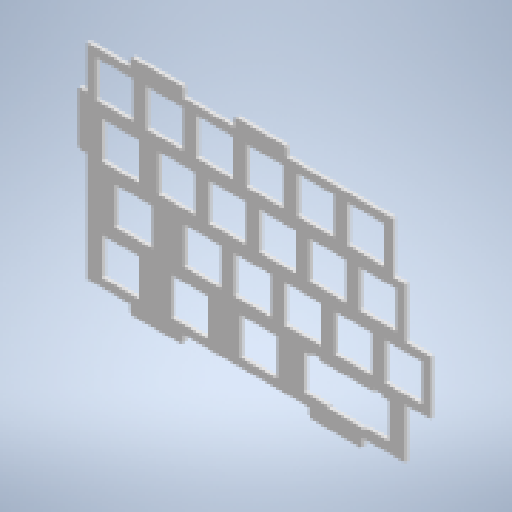
# Autodesk Inventor part: Plate_Left
Saved by Autodesk Inventor 2023 (Build 270158000, 158)
## iProperties
Created: 2022-11-13
Part Number: Plate_Left
Material: Generic
Document SubType Name: Modeling
Designer: reide
Density: 1 g/cm^3
Appearance: Default
Author: reide
Autodesk Inventor part; units mm, degrees
ref_plane "YZ Plane" through (0, 0, 0) normal (1, 0, 0) x (0, 1, 0)
ref_plane "XZ Plane" through (0, 0, 0) normal (0, 1, 0) x (-1, 0, 0)
ref_plane "XY Plane" through (0, 0, 0) normal (0, 0, 1) x (1, 0, 0)
sketch "Sketch1" plane through (0, 0, 0) normal (0, 0, 1) x (1, 0, 0)
  line L0 (115.8, 77.7) -> (0, 77.7)
  line L1 (0, 77.7) -> (0, 0)
  line L2 (0, 0) -> (120.562, 0)
  line L3 (120.562, 19.05) -> (120.562, 0)
  line L4 (130.0875, 19.05) -> (120.562, 19.05)
  line L5 (130.0875, 39.6) -> (130.0875, 19.05)
  line L6 (120.5625, 39.6) -> (130.0875, 39.6)
  line L7 (120.5625, 58.65) -> (120.5625, 39.6)
  line L8 (115.8, 58.65) -> (120.5625, 58.65)
  line L9 (115.8, 77.7) -> (115.8, 58.65)
  line L10 (10.4187, 22.325) -> (10.4187, 36.325)
  line L11 (10.4187, 36.325) -> (24.4187, 36.325)
  line L12 (24.4187, 36.325) -> (24.4187, 22.325)
  line L13 (24.4187, 22.325) -> (10.4187, 22.325)
  line L14 (58.0437, 3.275) -> (58.0437, 17.275)
  line L15 (58.0437, 17.275) -> (72.0437, 17.275)
  line L16 (72.0437, 17.275) -> (72.0437, 3.275)
  line L17 (72.0437, 3.275) -> (58.0437, 3.275)
  line L18 (31.85, 3.275) -> (31.85, 17.275)
  line L19 (31.85, 17.275) -> (45.85, 17.275)
  line L20 (45.85, 17.275) -> (45.85, 3.275)
  line L21 (45.85, 3.275) -> (31.85, 3.275)
  line L22 (5.6562, 3.275) -> (5.6562, 17.275)
  line L23 (5.6562, 17.275) -> (19.6562, 17.275)
  line L24 (19.6562, 17.275) -> (19.6562, 3.275)
  line L25 (19.6562, 3.275) -> (5.6562, 3.275)
  line L26 (5.6562, 41.375) -> (5.6562, 55.375)
  line L27 (5.6562, 55.375) -> (19.6562, 55.375)
  line L28 (19.6562, 55.375) -> (19.6562, 41.375)
  line L29 (19.6562, 41.375) -> (5.6562, 41.375)
  line L30 (112.8125, 22.325) -> (112.8125, 36.325)
  line L31 (112.8125, 36.325) -> (126.8125, 36.325)
  line L32 (126.8125, 36.325) -> (126.8125, 22.325)
  line L33 (126.8125, 22.325) -> (112.8125, 22.325)
  line L34 (93.7625, 22.325) -> (93.7625, 36.325)
  line L35 (93.7625, 36.325) -> (107.7625, 36.325)
  line L36 (107.7625, 36.325) -> (107.7625, 22.325)
  line L37 (107.7625, 22.325) -> (93.7625, 22.325)
  line L38 (74.7125, 22.325) -> (74.7125, 36.325)
  line L39 (74.7125, 36.325) -> (88.7125, 36.325)
  line L40 (88.7125, 36.325) -> (88.7125, 22.325)
  line L41 (88.7125, 22.325) -> (74.7125, 22.325)
  line L42 (55.6625, 22.325) -> (55.6625, 36.325)
  line L43 (55.6625, 36.325) -> (69.6625, 36.325)
  line L44 (69.6625, 36.325) -> (69.6625, 22.325)
  line L45 (69.6625, 22.325) -> (55.6625, 22.325)
  line L46 (36.6125, 22.325) -> (36.6125, 36.325)
  line L47 (36.6125, 36.325) -> (50.6125, 36.325)
  line L48 (50.6125, 36.325) -> (50.6125, 22.325)
  line L49 (50.6125, 22.325) -> (36.6125, 22.325)
  line L50 (103.2875, 41.375) -> (103.2875, 55.375)
  line L51 (103.2875, 55.375) -> (117.2875, 55.375)
  line L52 (117.2875, 55.375) -> (117.2875, 41.375)
  line L53 (117.2875, 41.375) -> (103.2875, 41.375)
  line L54 (84.2375, 41.375) -> (84.2375, 55.375)
  line L55 (84.2375, 55.375) -> (98.2375, 55.375)
  line L56 (98.2375, 55.375) -> (98.2375, 41.375)
  line L57 (98.2375, 41.375) -> (84.2375, 41.375)
  line L58 (65.1875, 41.375) -> (65.1875, 55.375)
  line L59 (65.1875, 55.375) -> (79.1875, 55.375)
  line L60 (79.1875, 55.375) -> (79.1875, 41.375)
  line L61 (79.1875, 41.375) -> (65.1875, 41.375)
  line L62 (46.1375, 41.375) -> (46.1375, 55.375)
  line L63 (46.1375, 55.375) -> (60.1375, 55.375)
  line L64 (60.1375, 55.375) -> (60.1375, 41.375)
  line L65 (60.1375, 41.375) -> (46.1375, 41.375)
  line L66 (27.0875, 41.375) -> (27.0875, 55.375)
  line L67 (27.0875, 55.375) -> (41.0875, 55.375)
  line L68 (41.0875, 55.375) -> (41.0875, 41.375)
  line L69 (41.0875, 41.375) -> (27.0875, 41.375)
  line L70 (98.525, 60.425) -> (98.525, 74.425)
  line L71 (98.525, 74.425) -> (112.525, 74.425)
  line L72 (112.525, 74.425) -> (112.525, 60.425)
  line L73 (112.525, 60.425) -> (98.525, 60.425)
  line L74 (79.475, 60.425) -> (79.475, 74.425)
  line L75 (79.475, 74.425) -> (93.475, 74.425)
  line L76 (93.475, 74.425) -> (93.475, 60.425)
  line L77 (93.475, 60.425) -> (79.475, 60.425)
  line L78 (60.425, 60.425) -> (60.425, 74.425)
  line L79 (60.425, 74.425) -> (74.425, 74.425)
  line L80 (74.425, 74.425) -> (74.425, 60.425)
  line L81 (74.425, 60.425) -> (60.425, 60.425)
  line L82 (41.375, 60.425) -> (41.375, 74.425)
  line L83 (41.375, 74.425) -> (55.375, 74.425)
  line L84 (55.375, 74.425) -> (55.375, 60.425)
  line L85 (55.375, 60.425) -> (41.375, 60.425)
  line L86 (22.325, 60.425) -> (22.325, 74.425)
  line L87 (22.325, 74.425) -> (36.325, 74.425)
  line L88 (36.325, 74.425) -> (36.325, 60.425)
  line L89 (36.325, 60.425) -> (22.325, 60.425)
  line L90 (3.275, 60.425) -> (3.275, 74.425)
  line L91 (3.275, 74.425) -> (17.275, 74.425)
  line L92 (17.275, 74.425) -> (17.275, 60.425)
  line L93 (17.275, 60.425) -> (3.275, 60.425)
  line L94 (88.1304, 17.275) -> (108.6315, 17.275)
  line L95 (108.6315, 17.275) -> (108.6315, 18.2451)
  line L96 (108.6315, 18.2451) -> (111.9306, 18.2451)
  line L97 (111.9306, 18.2451) -> (111.9306, 17.275)
  line L98 (111.9306, 17.275) -> (114.4058, 17.275)
  line L99 (114.4058, 17.275) -> (114.4059, 17.0334)
  line L100 (114.4059, 17.0334) -> (114.4058, 3.9957)
  line L101 (114.4058, 3.9957) -> (106.9062, 3.9957)
  line L102 (106.9062, 3.9957) -> (105.3807, 3.9957)
  line L103 (105.3807, 3.9957) -> (105.3807, 3.2757)
  line L104 (105.3807, 3.2757) -> (91.3812, 3.2757)
  line L105 (91.3812, 3.2757) -> (91.3812, 3.9957)
  line L106 (91.3812, 3.9957) -> (82.3562, 3.9957)
  line L107 (82.3562, 3.9957) -> (82.3562, 17.0464)
  line L108 (82.3562, 17.0464) -> (82.3562, 17.275)
  line L109 (82.3562, 17.275) -> (84.8314, 17.275)
  line L110 (84.8314, 17.275) -> (84.8314, 18.2451)
  line L111 (84.8314, 18.2451) -> (88.1304, 18.2451)
  line L112 (88.1304, 18.2451) -> (88.1304, 17.275)
  point P0 (0.75, 76.95)
  constraints: 226 end point
extrude "Extrusion1" add sketch "Sketch1" along normal blind 1.4
sketch "Sketch2" plane through (0, 0, 1.4) normal (0, 0, 1) x (1, 0, 0)
  line L0 (19.6562, 41.375) -> (5.6562, 41.375) projected
  line L1 (0, 77.7) -> (0, 0) projected
  line L2 (0, 41.375) -> (0, 61.375)
  line L3 (0, 61.375) -> (-3.5, 61.375)
  line L4 (-3.5, 61.375) -> (-3.5, 41.375)
  line L5 (-3.5, 41.375) -> (0, 41.375)
  arc A0 (77.3, 76.2) -> (81.3, 80.2) centre (77.3, 80.2) ccw projected
  line L6 (1.25, 76.2) -> (77.3, 76.2) projected
  line L7 (1.25, 41.0243) -> (1.25, 76.2) projected
  line L8 (-0.25, 41.0243) -> (1.25, 41.0243) projected
  line L9 (-0.25, 41.0243) -> (-0.25, 33.75) projected
  line L10 (-0.25, 33.75) -> (-1.25, 33.75) projected
  line L11 (-1.25, 33.75) -> (-1.25, 35.75) projected
  line L12 (-1.25, 35.75) -> (-5.25, 35.75) projected
  line L13 (-5.25, 35.75) -> (-5.25, 81.45) projected
  arc A1 (-2.25, 84.45) -> (-5.25, 81.45) centre (-2.25, 81.45) ccw projected
  line L14 (85.05, 84.45) -> (-2.25, 84.45) projected
  line L15 (85.05, 83.45) -> (85.05, 84.45) projected
  line L16 (81.3, 83.45) -> (85.05, 83.45) projected
  line L17 (81.3, 80.2) -> (81.3, 83.45) projected
  circle A2 centre (63.044, 80.2) radius 1.5 projected
  circle A3 centre (-1, 80.2) radius 1.5 projected
  circle A4 centre (-1.75, 49.45) radius 1.5 projected
  line L18 (117.025, 56.875) -> (117.7875, 56.875) projected
  line L19 (117.7875, 56.875) -> (117.7875, 41.825) projected
  arc A5 (117.7875, 41.825) -> (121.7875, 37.825) centre (121.7875, 41.825) ccw projected
  line L20 (121.7875, 37.825) -> (116.8125, 37.825) projected
  line L21 (116.8125, 37.825) -> (116.8125, 36.325) projected
  line L22 (116.8125, 36.325) -> (112.8125, 36.325) projected
  line L23 (112.8125, 36.325) -> (112.8125, 22.325) projected
  line L24 (112.8125, 22.325) -> (107.7625, 22.325) projected
  line L25 (107.7625, 22.325) -> (107.7625, 36.325) projected
  line L26 (107.7625, 36.325) -> (103.7625, 36.325) projected
  line L27 (103.7625, 36.325) -> (103.7625, 37.825) projected
  line L28 (103.7625, 37.825) -> (97.7625, 37.825) projected
  line L29 (97.7625, 37.825) -> (97.7625, 36.325) projected
  line L30 (97.7625, 36.325) -> (93.7625, 36.325) projected
  line L31 (93.7625, 36.325) -> (93.7625, 22.325) projected
  line L32 (93.7625, 22.325) -> (88.7125, 22.325) projected
  line L33 (88.7125, 22.325) -> (88.7125, 36.325) projected
  line L34 (88.7125, 36.325) -> (84.7125, 36.325) projected
  line L35 (84.7125, 36.325) -> (84.7125, 37.825) projected
  line L36 (84.7125, 37.825) -> (78.7125, 37.825) projected
  line L37 (78.7125, 37.825) -> (78.7125, 36.325) projected
  line L38 (78.7125, 36.325) -> (74.7125, 36.325) projected
  line L39 (74.7125, 36.325) -> (74.7125, 22.325) projected
  line L40 (74.7125, 22.325) -> (78.7125, 22.325) projected
  line L41 (78.7125, 22.325) -> (78.7125, 20.825) projected
  line L42 (78.7125, 20.825) -> (83.1062, 20.825) projected
  line L43 (83.1062, 20.825) -> (83.1062, 17.275) projected
  line L44 (83.1062, 17.275) -> (82.3562, 17.275) projected
  line L45 (82.3562, 17.275) -> (82.3562, 17.0464) projected
  line L46 (82.3562, 17.0464) -> (82.3562, 3.9957) projected
  line L47 (82.3562, 3.9957) -> (83.1062, 3.9957) projected
  line L48 (83.1062, 3.9957) -> (83.1062, 1.5) projected
  line L49 (83.1062, 1.5) -> (1.25, 1.5) projected
  line L50 (1.25, 1.5) -> (1.25, 18.4694) projected
  line L51 (1.25, 18.4694) -> (-0.25, 18.4694) projected
  line L52 (-0.25, 41.0243) -> (-0.25, 18.4694) projected
  line L53 (-0.25, 41.0243) -> (1.25, 41.0243) projected
  line L54 (1.25, 41.0243) -> (1.25, 76.2) projected
  line L55 (1.25, 76.2) -> (77.3, 76.2) projected
  arc A6 (77.3, 76.2) -> (81.3, 80.2) centre (77.3, 80.2) ccw projected
  line L56 (81.3, 80.2) -> (81.3, 83.45) projected
  line L57 (81.3, 83.45) -> (99.3, 83.45) projected
  line L58 (99.3, 83.45) -> (99.3, 80.2) projected
  arc A7 (99.3, 80.2) -> (103.3, 76.2) centre (103.3, 80.2) ccw projected
  line L59 (103.3, 76.2) -> (113.025, 76.2) projected
  line L60 (113.025, 76.2) -> (113.025, 60.875) projected
  arc A8 (113.025, 60.875) -> (117.025, 56.875) centre (117.025, 60.875) ccw projected
  line L61 (113.2875, 56.875) -> (107.2875, 56.875) projected
  line L62 (107.2875, 56.875) -> (107.2875, 55.375) projected
  line L63 (107.2875, 55.375) -> (103.2875, 55.375) projected
  line L64 (103.2875, 55.375) -> (103.2875, 41.375) projected
  line L65 (103.2875, 41.375) -> (107.2875, 41.375) projected
  line L66 (107.2875, 41.375) -> (107.2875, 39.875) projected
  line L67 (107.2875, 39.875) -> (113.2875, 39.875) projected
  line L68 (113.2875, 39.875) -> (113.2875, 41.375) projected
  line L69 (113.2875, 41.375) -> (117.2875, 41.375) projected
  line L70 (117.2875, 41.375) -> (117.2875, 55.375) projected
  line L71 (117.2875, 55.375) -> (113.2875, 55.375) projected
  line L72 (113.2875, 55.375) -> (113.2875, 56.875) projected
  line L73 (13.275, 58.925) -> (13.275, 60.425) projected
  line L74 (13.275, 60.425) -> (17.275, 60.425) projected
  line L75 (17.275, 60.425) -> (17.275, 74.425) projected
  line L76 (17.275, 74.425) -> (13.275, 74.425) projected
  line L77 (13.275, 74.425) -> (13.275, 75.925) projected
  line L78 (13.275, 75.925) -> (7.275, 75.925) projected
  line L79 (7.275, 75.925) -> (7.275, 74.425) projected
  line L80 (7.275, 74.425) -> (3.275, 74.425) projected
  line L81 (3.275, 74.425) -> (3.275, 60.425) projected
  line L82 (3.275, 60.425) -> (7.275, 60.425) projected
  line L83 (7.275, 60.425) -> (7.275, 58.925) projected
  line L84 (7.275, 58.925) -> (13.275, 58.925) projected
  line L85 (32.325, 58.925) -> (32.325, 60.425) projected
  line L86 (32.325, 60.425) -> (36.325, 60.425) projected
  line L87 (36.325, 60.425) -> (36.325, 74.425) projected
  line L88 (36.325, 74.425) -> (32.325, 74.425) projected
  line L89 (32.325, 74.425) -> (32.325, 75.925) projected
  line L90 (32.325, 75.925) -> (26.325, 75.925) projected
  line L91 (26.325, 75.925) -> (26.325, 74.425) projected
  line L92 (26.325, 74.425) -> (22.325, 74.425) projected
  line L93 (22.325, 74.425) -> (22.325, 60.425) projected
  line L94 (22.325, 60.425) -> (26.325, 60.425) projected
  line L95 (26.325, 60.425) -> (26.325, 58.925) projected
  line L96 (26.325, 58.925) -> (32.325, 58.925) projected
  line L97 (51.375, 58.925) -> (51.375, 60.425) projected
  line L98 (51.375, 60.425) -> (55.375, 60.425) projected
  line L99 (55.375, 60.425) -> (55.375, 74.425) projected
  line L100 (55.375, 74.425) -> (51.375, 74.425) projected
  line L101 (51.375, 74.425) -> (51.375, 75.925) projected
  line L102 (51.375, 75.925) -> (45.375, 75.925) projected
  line L103 (45.375, 75.925) -> (45.375, 74.425) projected
  line L104 (45.375, 74.425) -> (41.375, 74.425) projected
  line L105 (41.375, 74.425) -> (41.375, 60.425) projected
  line L106 (41.375, 60.425) -> (45.375, 60.425) projected
  line L107 (45.375, 60.425) -> (45.375, 58.925) projected
  line L108 (45.375, 58.925) -> (51.375, 58.925) projected
  line L109 (70.425, 58.925) -> (70.425, 60.425) projected
  line L110 (70.425, 60.425) -> (74.425, 60.425) projected
  line L111 (74.425, 60.425) -> (74.425, 74.425) projected
  line L112 (74.425, 74.425) -> (70.425, 74.425) projected
  line L113 (70.425, 74.425) -> (70.425, 75.925) projected
  line L114 (70.425, 75.925) -> (64.425, 75.925) projected
  line L115 (64.425, 75.925) -> (64.425, 74.425) projected
  line L116 (64.425, 74.425) -> (60.425, 74.425) projected
  line L117 (60.425, 74.425) -> (60.425, 60.425) projected
  line L118 (60.425, 60.425) -> (64.425, 60.425) projected
  line L119 (64.425, 60.425) -> (64.425, 58.925) projected
  line L120 (64.425, 58.925) -> (70.425, 58.925) projected
  line L121 (89.475, 58.925) -> (89.475, 60.425) projected
  line L122 (89.475, 60.425) -> (93.475, 60.425) projected
  line L123 (93.475, 60.425) -> (93.475, 74.425) projected
  line L124 (93.475, 74.425) -> (89.475, 74.425) projected
  line L125 (89.475, 74.425) -> (89.475, 75.925) projected
  line L126 (89.475, 75.925) -> (83.475, 75.925) projected
  line L127 (83.475, 75.925) -> (83.475, 74.425) projected
  line L128 (83.475, 74.425) -> (79.475, 74.425) projected
  line L129 (79.475, 74.425) -> (79.475, 60.425) projected
  line L130 (79.475, 60.425) -> (83.475, 60.425) projected
  line L131 (83.475, 60.425) -> (83.475, 58.925) projected
  line L132 (83.475, 58.925) -> (89.475, 58.925) projected
  line L133 (108.525, 58.925) -> (108.525, 60.425) projected
  line L134 (108.525, 60.425) -> (112.525, 60.425) projected
  line L135 (112.525, 60.425) -> (112.525, 74.425) projected
  line L136 (112.525, 74.425) -> (108.525, 74.425) projected
  line L137 (108.525, 74.425) -> (108.525, 75.925) projected
  line L138 (108.525, 75.925) -> (102.525, 75.925) projected
  line L139 (102.525, 75.925) -> (102.525, 74.425) projected
  line L140 (102.525, 74.425) -> (98.525, 74.425) projected
  line L141 (98.525, 74.425) -> (98.525, 60.425) projected
  line L142 (98.525, 60.425) -> (102.525, 60.425) projected
  line L143 (102.525, 60.425) -> (102.525, 58.925) projected
  line L144 (102.525, 58.925) -> (108.525, 58.925) projected
  line L145 (37.0875, 39.875) -> (37.0875, 41.375) projected
  line L146 (37.0875, 41.375) -> (41.0875, 41.375) projected
  line L147 (41.0875, 41.375) -> (41.0875, 55.375) projected
  line L148 (41.0875, 55.375) -> (37.0875, 55.375) projected
  line L149 (37.0875, 55.375) -> (37.0875, 56.875) projected
  line L150 (37.0875, 56.875) -> (31.0875, 56.875) projected
  line L151 (31.0875, 56.875) -> (31.0875, 55.375) projected
  line L152 (31.0875, 55.375) -> (27.0875, 55.375) projected
  line L153 (27.0875, 55.375) -> (27.0875, 41.375) projected
  line L154 (27.0875, 41.375) -> (31.0875, 41.375) projected
  line L155 (31.0875, 41.375) -> (31.0875, 39.875) projected
  line L156 (31.0875, 39.875) -> (37.0875, 39.875) projected
  line L157 (50.1375, 56.875) -> (50.1375, 55.375) projected
  line L158 (50.1375, 55.375) -> (46.1375, 55.375) projected
  line L159 (46.1375, 55.375) -> (46.1375, 41.375) projected
  line L160 (46.1375, 41.375) -> (50.1375, 41.375) projected
  line L161 (50.1375, 41.375) -> (50.1375, 39.875) projected
  line L162 (50.1375, 39.875) -> (56.1375, 39.875) projected
  line L163 (56.1375, 39.875) -> (56.1375, 41.375) projected
  line L164 (56.1375, 41.375) -> (60.1375, 41.375) projected
  line L165 (60.1375, 41.375) -> (60.1375, 55.375) projected
  line L166 (60.1375, 55.375) -> (56.1375, 55.375) projected
  line L167 (56.1375, 55.375) -> (56.1375, 56.875) projected
  line L168 (56.1375, 56.875) -> (50.1375, 56.875) projected
  line L169 (69.1875, 56.875) -> (69.1875, 55.375) projected
  line L170 (69.1875, 55.375) -> (65.1875, 55.375) projected
  line L171 (65.1875, 55.375) -> (65.1875, 41.375) projected
  line L172 (65.1875, 41.375) -> (69.1875, 41.375) projected
  line L173 (69.1875, 41.375) -> (69.1875, 39.875) projected
  line L174 (69.1875, 39.875) -> (75.1875, 39.875) projected
  line L175 (75.1875, 39.875) -> (75.1875, 41.375) projected
  line L176 (75.1875, 41.375) -> (79.1875, 41.375) projected
  line L177 (79.1875, 41.375) -> (79.1875, 55.375) projected
  line L178 (79.1875, 55.375) -> (75.1875, 55.375) projected
  line L179 (75.1875, 55.375) -> (75.1875, 56.875) projected
  line L180 (75.1875, 56.875) -> (69.1875, 56.875) projected
  line L181 (88.2375, 56.875) -> (88.2375, 55.375) projected
  line L182 (88.2375, 55.375) -> (84.2375, 55.375) projected
  line L183 (84.2375, 55.375) -> (84.2375, 41.375) projected
  line L184 (84.2375, 41.375) -> (88.2375, 41.375) projected
  line L185 (88.2375, 41.375) -> (88.2375, 39.875) projected
  line L186 (88.2375, 39.875) -> (94.2375, 39.875) projected
  line L187 (94.2375, 39.875) -> (94.2375, 41.375) projected
  line L188 (94.2375, 41.375) -> (98.2375, 41.375) projected
  line L189 (98.2375, 41.375) -> (98.2375, 55.375) projected
  line L190 (98.2375, 55.375) -> (94.2375, 55.375) projected
  line L191 (94.2375, 55.375) -> (94.2375, 56.875) projected
  line L192 (94.2375, 56.875) -> (88.2375, 56.875) projected
  line L193 (46.6125, 20.825) -> (46.6125, 22.325) projected
  line L194 (46.6125, 22.325) -> (50.6125, 22.325) projected
  line L195 (50.6125, 22.325) -> (50.6125, 36.325) projected
  line L196 (50.6125, 36.325) -> (46.6125, 36.325) projected
  line L197 (46.6125, 36.325) -> (46.6125, 37.825) projected
  line L198 (46.6125, 37.825) -> (40.6125, 37.825) projected
  line L199 (40.6125, 37.825) -> (40.6125, 36.325) projected
  line L200 (40.6125, 36.325) -> (36.6125, 36.325) projected
  line L201 (36.6125, 36.325) -> (36.6125, 22.325) projected
  line L202 (36.6125, 22.325) -> (40.6125, 22.325) projected
  line L203 (40.6125, 22.325) -> (40.6125, 20.825) projected
  line L204 (40.6125, 20.825) -> (46.6125, 20.825) projected
  line L205 (65.6625, 20.825) -> (65.6625, 22.325) projected
  line L206 (65.6625, 22.325) -> (69.6625, 22.325) projected
  line L207 (69.6625, 22.325) -> (69.6625, 36.325) projected
  line L208 (69.6625, 36.325) -> (65.6625, 36.325) projected
  line L209 (65.6625, 36.325) -> (65.6625, 37.825) projected
  line L210 (65.6625, 37.825) -> (59.6625, 37.825) projected
  line L211 (59.6625, 37.825) -> (59.6625, 36.325) projected
  line L212 (59.6625, 36.325) -> (55.6625, 36.325) projected
  line L213 (55.6625, 36.325) -> (55.6625, 22.325) projected
  line L214 (55.6625, 22.325) -> (59.6625, 22.325) projected
  line L215 (59.6625, 22.325) -> (59.6625, 20.825) projected
  line L216 (59.6625, 20.825) -> (65.6625, 20.825) projected
  line L217 (15.6562, 39.875) -> (15.6562, 41.375) projected
  line L218 (15.6562, 41.375) -> (19.6562, 41.375) projected
  line L219 (19.6562, 41.375) -> (19.6562, 55.375) projected
  line L220 (19.6562, 55.375) -> (15.6562, 55.375) projected
  line L221 (15.6562, 55.375) -> (15.6562, 56.875) projected
  line L222 (15.6562, 56.875) -> (9.6562, 56.875) projected
  line L223 (9.6562, 56.875) -> (9.6562, 55.375) projected
  line L224 (9.6562, 55.375) -> (5.6562, 55.375) projected
  line L225 (5.6562, 55.375) -> (5.6562, 41.375) projected
  line L226 (5.6562, 41.375) -> (9.6562, 41.375) projected
  line L227 (9.6562, 41.375) -> (9.6562, 39.875) projected
  line L228 (9.6562, 39.875) -> (15.6562, 39.875) projected
  line L229 (20.4187, 20.825) -> (20.4187, 22.325) projected
  line L230 (20.4187, 22.325) -> (24.4187, 22.325) projected
  line L231 (24.4187, 22.325) -> (24.4187, 36.325) projected
  line L232 (24.4187, 36.325) -> (20.4187, 36.325) projected
  line L233 (20.4187, 36.325) -> (20.4187, 37.825) projected
  line L234 (20.4187, 37.825) -> (14.4187, 37.825) projected
  line L235 (14.4187, 37.825) -> (14.4187, 36.325) projected
  line L236 (14.4187, 36.325) -> (10.4187, 36.325) projected
  line L237 (10.4187, 36.325) -> (10.4187, 22.325) projected
  line L238 (10.4187, 22.325) -> (14.4187, 22.325) projected
  line L239 (14.4187, 22.325) -> (14.4187, 20.825) projected
  line L240 (14.4187, 20.825) -> (20.4187, 20.825) projected
  line L241 (15.6562, 1.775) -> (15.6562, 3.275) projected
  line L242 (15.6562, 3.275) -> (19.6562, 3.275) projected
  line L243 (19.6562, 3.275) -> (19.6562, 17.275) projected
  line L244 (19.6562, 17.275) -> (15.6562, 17.275) projected
  line L245 (15.6562, 17.275) -> (15.6562, 18.775) projected
  line L246 (15.6562, 18.775) -> (9.6562, 18.775) projected
  line L247 (9.6562, 18.775) -> (9.6562, 17.275) projected
  line L248 (9.6562, 17.275) -> (5.6562, 17.275) projected
  line L249 (5.6562, 17.275) -> (5.6562, 3.275) projected
  line L250 (5.6562, 3.275) -> (9.6562, 3.275) projected
  line L251 (9.6562, 3.275) -> (9.6562, 1.775) projected
  line L252 (9.6562, 1.775) -> (15.6562, 1.775) projected
  line L253 (41.85, 1.775) -> (41.85, 3.275) projected
  line L254 (41.85, 3.275) -> (45.85, 3.275) projected
  line L255 (45.85, 3.275) -> (45.85, 17.275) projected
  line L256 (45.85, 17.275) -> (41.85, 17.275) projected
  line L257 (41.85, 17.275) -> (41.85, 18.775) projected
  line L258 (41.85, 18.775) -> (35.85, 18.775) projected
  line L259 (35.85, 18.775) -> (35.85, 17.275) projected
  line L260 (35.85, 17.275) -> (31.85, 17.275) projected
  line L261 (31.85, 17.275) -> (31.85, 3.275) projected
  line L262 (31.85, 3.275) -> (35.85, 3.275) projected
  line L263 (35.85, 3.275) -> (35.85, 1.775) projected
  line L264 (35.85, 1.775) -> (41.85, 1.775) projected
  line L265 (68.0437, 1.775) -> (68.0437, 3.275) projected
  line L266 (68.0437, 3.275) -> (72.0437, 3.275) projected
  line L267 (72.0437, 3.275) -> (72.0437, 17.275) projected
  line L268 (72.0437, 17.275) -> (68.0437, 17.275) projected
  line L269 (68.0437, 17.275) -> (68.0437, 18.775) projected
  line L270 (68.0437, 18.775) -> (62.0437, 18.775) projected
  line L271 (62.0437, 18.775) -> (62.0437, 17.275) projected
  line L272 (62.0437, 17.275) -> (58.0437, 17.275) projected
  line L273 (58.0437, 17.275) -> (58.0437, 3.275) projected
  line L274 (58.0437, 3.275) -> (62.0437, 3.275) projected
  line L275 (62.0437, 3.275) -> (62.0437, 1.775) projected
  line L276 (62.0437, 1.775) -> (68.0437, 1.775) projected
  arc A9 (99.3, 80.2) -> (103.3, 76.2) centre (103.3, 80.2) ccw projected
  line L277 (99.3, 84.45) -> (99.3, 80.2) projected
  line L278 (99.3, 84.45) -> (131.3375, 84.45) projected
  line L279 (131.3375, 84.45) -> (131.3375, -5.25) projected
  line L280 (131.3375, -5.25) -> (-2.25, -5.25) projected
  arc A10 (-5.25, -2.25) -> (-2.25, -5.25) centre (-2.25, -2.25) ccw projected
  line L281 (-5.25, -2.25) -> (-5.25, 22.75) projected
  line L282 (-5.25, 22.75) -> (-1.25, 22.75) projected
  line L283 (-1.25, 22.75) -> (-1.25, 24.75) projected
  line L284 (-1.25, 24.75) -> (-0.25, 24.75) projected
  line L285 (-0.25, 24.75) -> (-0.25, 18.4694) projected
  line L286 (1.25, 18.4694) -> (-0.25, 18.4694) projected
  line L287 (1.25, 1.5) -> (1.25, 18.4694) projected
  line L288 (83.1062, 1.5) -> (1.25, 1.5) projected
  line L289 (83.1062, -0.25) -> (83.1062, 1.5) projected
  line L290 (83.1062, -0.25) -> (113.6558, -0.25) projected
  line L291 (113.6558, 1.5) -> (113.6558, -0.25) projected
  line L292 (117.787, 1.5) -> (113.6558, 1.5) projected
  line L293 (117.787, 16.825) -> (117.787, 1.5) projected
  arc A11 (121.787, 20.825) -> (117.787, 16.825) centre (121.787, 16.825) ccw projected
  line L294 (127.3125, 20.825) -> (121.787, 20.825) projected
  line L295 (127.3125, 37.825) -> (127.3125, 20.825) projected
  line L296 (121.7875, 37.825) -> (127.3125, 37.825) projected
  arc A12 (117.7875, 41.825) -> (121.7875, 37.825) centre (121.7875, 41.825) ccw projected
  line L297 (117.7875, 56.875) -> (117.7875, 41.825) projected
  line L298 (117.025, 56.875) -> (117.7875, 56.875) projected
  arc A13 (113.025, 60.875) -> (117.025, 56.875) centre (117.025, 60.875) ccw projected
  line L299 (113.025, 76.2) -> (113.025, 60.875) projected
  line L300 (103.3, 76.2) -> (113.025, 76.2) projected
  circle A14 centre (127.0875, 80.2) radius 1.5 projected
  circle A15 centre (63.044, -1.75) radius 1.5 projected
  circle A16 centre (-1.75, -1.75) radius 1.5 projected
  circle A17 centre (127.0875, -1) radius 1.5 projected
  circle A18 centre (127.0875, 44.45) radius 1.5 projected
  line L301 (115.8, 77.7) -> (0, 77.7) projected
  line L302 (36.325, 77.7) -> (16.325, 77.7)
  line L303 (16.325, 77.7) -> (16.325, 81.2)
  line L304 (16.325, 81.2) -> (36.325, 81.2)
  line L305 (36.325, 81.2) -> (36.325, 77.7)
  line L306 (55.6625, 77.7) -> (75.6625, 77.7)
  line L307 (75.6625, 77.7) -> (75.6625, 81.2)
  line L308 (75.6625, 81.2) -> (55.6625, 81.2)
  line L309 (55.6625, 81.2) -> (55.6625, 77.7)
  line L310 (0, 0) -> (120.562, 0) projected
  line L311 (16.325, 0) -> (36.325, 0)
  line L312 (16.325, 0) -> (16.325, -3.5)
  line L313 (16.325, -3.5) -> (36.325, -3.5)
  line L314 (36.325, -3.5) -> (36.325, 0)
  line L315 (60.281, 0) -> (60.281, -3.5)
  line L316 (-10.7755, -5.25) -> (122.812, -5.25)
  line L317 (118.562, 0) -> (2, 0)
  line L318 (104.237, 0) -> (84.237, 0)
  line L319 (104.237, 0) -> (104.237, -3.5)
  line L320 (104.237, -3.5) -> (84.237, -3.5)
  line L321 (84.237, -3.5) -> (84.237, 0)
  point P0 (0, 75.7)
  point P1 (0, 2)
  point P2 (113.8, 77.7)
  point P3 (2, 77.7)
  point P4 (2, 0)
  point P5 (104.237, -0.25)
  point P6 (84.237, -0.25)
  dimension "d3" = 20
  dimension "d4" = 3.5
  dimension "d5" = 20
  dimension "d6" = 3.5
  dimension "d7" = 20
  dimension "d8" = 3.5
  constraints: 46 end point, 14 point on line, 10 perpendicular, 8 symmetric about line, 1 horizontal, 1 midpoint, 1 vertical
  measures "d3" distance of L2.start L2.end
  measures "d4" distance of L2.end L3.end
  measures "d5" distance of L302.start L302.end
  measures "d6" distance of L302.end L303.end
  measures "d7" distance of L306.start L306.end
  measures "d8" distance of L311.start L312.end
extrude "Extrusion2" add sketch "Sketch2" against normal blind 1.4 contours L1 L5 L4 L3 | L303 L304 L305 L301 | L309 L308 A2 L307 L301 | L308 A2 | L310 L314 L313 L312 | L310 L319 L290 L321 | L290 L319 L320 L321 | A4 picked at (62.9827, 80.3704)
fillet "Fillet2" radius 1 10 edges at (16.325, 81.2, 0.7) (36.325, 81.2, 0.7) (55.6625, 81.2, 0.7) (75.6625, 81.2, 0.7) (-3.5, 61.375, 0.7) (-3.5, 41.375, 0.7) (16.325, -3.5, 0.7) (36.325, -3.5, 0.7) (84.237, -3.5, 0.7) (104.237, -3.5, 0.7)
sketch "Sketch3" plane through (0, 0, 1.4) normal (0, 0, 1) x (1, 0, 0)
  line L0 (132.4924, 17.275) -> (152.9935, 17.275) projected
  line L1 (152.9935, 17.275) -> (152.9935, 18.2451) projected
  line L2 (152.9935, 18.2451) -> (156.2926, 18.2451) projected
  line L3 (156.2926, 18.2451) -> (156.2926, 17.275) projected
  line L4 (156.2926, 17.275) -> (158.7678, 17.275) projected
  line L5 (158.7678, 17.275) -> (158.7678, 3.9957) projected
  line L6 (158.7678, 3.9957) -> (149.7427, 3.9957) projected
  line L7 (149.7427, 3.9957) -> (149.7427, 3.2757) projected
  line L8 (149.7427, 3.2757) -> (135.7432, 3.2757) projected
  line L9 (135.7432, 3.2757) -> (135.7432, 3.9957) projected
  line L10 (135.7432, 3.9957) -> (126.7182, 3.9957) projected
  line L11 (126.7182, 3.9957) -> (126.7182, 17.275) projected
  line L12 (126.7182, 17.275) -> (129.1934, 17.275) projected
  line L13 (129.1934, 17.275) -> (129.1934, 18.2451) projected
  line L14 (129.1934, 18.2451) -> (132.4924, 18.2451) projected
  line L15 (132.4924, 18.2451) -> (132.4924, 17.275) projected
  line L16 (119.0745, 60.425) -> (119.0745, 74.425) projected
  line L17 (119.0745, 74.425) -> (133.0745, 74.425) projected
  line L18 (133.0745, 74.425) -> (133.0745, 60.425) projected
  line L19 (133.0745, 60.425) -> (119.0745, 60.425) projected
  line L20 (138.1245, 60.425) -> (138.1245, 74.425) projected
  line L21 (138.1245, 74.425) -> (152.1245, 74.425) projected
  line L22 (152.1245, 74.425) -> (152.1245, 60.425) projected
  line L23 (152.1245, 60.425) -> (138.1245, 60.425) projected
  line L24 (157.1745, 60.425) -> (157.1745, 74.425) projected
  line L25 (157.1745, 74.425) -> (171.1745, 74.425) projected
  line L26 (171.1745, 74.425) -> (171.1745, 60.425) projected
  line L27 (171.1745, 60.425) -> (157.1745, 60.425) projected
  line L28 (176.2245, 60.425) -> (176.2245, 74.425) projected
  line L29 (176.2245, 74.425) -> (190.2245, 74.425) projected
  line L30 (190.2245, 74.425) -> (190.2245, 60.425) projected
  line L31 (190.2245, 60.425) -> (176.2245, 60.425) projected
  line L32 (195.2745, 60.425) -> (195.2745, 74.425) projected
  line L33 (195.2745, 74.425) -> (209.2745, 74.425) projected
  line L34 (209.2745, 74.425) -> (209.2745, 60.425) projected
  line L35 (209.2745, 60.425) -> (195.2745, 60.425) projected
  line L36 (214.3245, 60.425) -> (214.3245, 74.425) projected
  line L37 (214.3245, 74.425) -> (228.3245, 74.425) projected
  line L38 (228.3245, 74.425) -> (228.3245, 60.425) projected
  line L39 (228.3245, 60.425) -> (214.3245, 60.425) projected
  line L40 (233.3745, 60.425) -> (233.3745, 74.425) projected
  line L41 (233.3745, 74.425) -> (247.3745, 74.425) projected
  line L42 (247.3745, 74.425) -> (247.3745, 60.425) projected
  line L43 (247.3745, 60.425) -> (233.3745, 60.425) projected
  line L44 (123.837, 41.375) -> (123.837, 55.375) projected
  line L45 (123.837, 55.375) -> (137.837, 55.375) projected
  line L46 (137.837, 55.375) -> (137.837, 41.375) projected
  line L47 (137.837, 41.375) -> (123.837, 41.375) projected
  line L48 (142.887, 41.375) -> (142.887, 55.375) projected
  line L49 (142.887, 55.375) -> (156.887, 55.375) projected
  line L50 (156.887, 55.375) -> (156.887, 41.375) projected
  line L51 (156.887, 41.375) -> (142.887, 41.375) projected
  line L52 (161.937, 41.375) -> (161.937, 55.375) projected
  line L53 (161.937, 55.375) -> (175.937, 55.375) projected
  line L54 (175.937, 55.375) -> (175.937, 41.375) projected
  line L55 (175.937, 41.375) -> (161.937, 41.375) projected
  line L56 (180.987, 41.375) -> (180.987, 55.375) projected
  line L57 (180.987, 55.375) -> (194.987, 55.375) projected
  line L58 (194.987, 55.375) -> (194.987, 41.375) projected
  line L59 (194.987, 41.375) -> (180.987, 41.375) projected
  line L60 (200.037, 41.375) -> (200.037, 55.375) projected
  line L61 (200.037, 55.375) -> (214.037, 55.375) projected
  line L62 (214.037, 55.375) -> (214.037, 41.375) projected
  line L63 (214.037, 41.375) -> (200.037, 41.375) projected
  line L64 (133.362, 22.325) -> (133.362, 36.325) projected
  line L65 (133.362, 36.325) -> (147.362, 36.325) projected
  line L66 (147.362, 36.325) -> (147.362, 22.325) projected
  line L67 (147.362, 22.325) -> (133.362, 22.325) projected
  line L68 (152.412, 22.325) -> (152.412, 36.325) projected
  line L69 (152.412, 36.325) -> (166.412, 36.325) projected
  line L70 (166.412, 36.325) -> (166.412, 22.325) projected
  line L71 (166.412, 22.325) -> (152.412, 22.325) projected
  line L72 (171.462, 22.325) -> (171.462, 36.325) projected
  line L73 (171.462, 36.325) -> (185.462, 36.325) projected
  line L74 (185.462, 36.325) -> (185.462, 22.325) projected
  line L75 (185.462, 22.325) -> (171.462, 22.325) projected
  line L76 (190.512, 22.325) -> (190.512, 36.325) projected
  line L77 (190.512, 36.325) -> (204.512, 36.325) projected
  line L78 (204.512, 36.325) -> (204.512, 22.325) projected
  line L79 (204.512, 22.325) -> (190.512, 22.325) projected
  line L80 (209.562, 22.325) -> (209.562, 36.325) projected
  line L81 (209.562, 36.325) -> (223.562, 36.325) projected
  line L82 (223.562, 36.325) -> (223.562, 22.325) projected
  line L83 (223.562, 22.325) -> (209.562, 22.325) projected
  line L84 (226.2307, 41.375) -> (226.2307, 55.375) projected
  line L85 (226.2307, 55.375) -> (240.2307, 55.375) projected
  line L86 (240.2307, 55.375) -> (240.2307, 41.375) projected
  line L87 (240.2307, 41.375) -> (226.2307, 41.375) projected
  line L88 (230.9932, 22.325) -> (230.9932, 36.325) projected
  line L89 (230.9932, 36.325) -> (244.9932, 36.325) projected
  line L90 (244.9932, 36.325) -> (244.9932, 22.325) projected
  line L91 (244.9932, 22.325) -> (230.9932, 22.325) projected
  line L92 (230.9932, 3.275) -> (230.9932, 17.275) projected
  line L93 (230.9932, 17.275) -> (244.9932, 17.275) projected
  line L94 (244.9932, 17.275) -> (244.9932, 3.275) projected
  line L95 (244.9932, 3.275) -> (230.9932, 3.275) projected
  line L96 (169.0807, 3.275) -> (169.0807, 17.275) projected
  line L97 (169.0807, 17.275) -> (183.0807, 17.275) projected
  line L98 (183.0807, 17.275) -> (183.0807, 3.275) projected
  line L99 (183.0807, 3.275) -> (169.0807, 3.275) projected
  line L100 (190.512, 3.275) -> (190.512, 17.275) projected
  line L101 (190.512, 17.275) -> (204.512, 17.275) projected
  line L102 (204.512, 17.275) -> (204.512, 3.275) projected
  line L103 (204.512, 3.275) -> (190.512, 3.275) projected
  line L104 (209.562, 3.275) -> (209.562, 17.275) projected
  line L105 (209.562, 17.275) -> (223.562, 17.275) projected
  line L106 (223.562, 17.275) -> (223.562, 3.275) projected
  line L107 (223.562, 3.275) -> (209.562, 3.275) projected
  line L108 (115.7995, 57.9) -> (120.5625, 57.9) projected
  line L109 (120.5625, 57.9) -> (120.5625, 39.6) projected
  line L110 (120.5625, 39.6) -> (120.562, 38.85) projected
  line L111 (120.562, 38.85) -> (130.0875, 38.85) projected
  line L112 (130.0875, 38.85) -> (130.0875, 19.8) projected
  line L113 (130.0875, 19.8) -> (120.562, 19.8) projected
  line L114 (120.562, 19.8) -> (120.562, 0) projected
  line L115 (120.562, 0) -> (136.887, 0) projected
  line L116 (136.887, 0) -> (136.887, -2.5) projected
  arc A0 (136.887, -2.5) -> (137.887, -3.5) centre (137.887, -2.5) ccw projected
  line L117 (137.887, -3.5) -> (155.887, -3.5) projected
  arc A1 (155.887, -3.5) -> (156.887, -2.5) centre (155.887, -2.5) ccw projected
  line L118 (156.887, -2.5) -> (156.887, 0) projected
  line L119 (156.887, 0) -> (214.3245, 0) projected
  line L120 (214.3245, 0) -> (214.3245, -2.5) projected
  arc A2 (214.3245, -2.5) -> (215.3245, -3.5) centre (215.3245, -2.5) ccw projected
  line L121 (215.3245, -3.5) -> (233.3245, -3.5) projected
  arc A3 (233.3245, -3.5) -> (234.3245, -2.5) centre (233.3245, -2.5) ccw projected
  line L122 (234.3245, -2.5) -> (234.3245, 0) projected
  line L123 (234.3245, 0) -> (250.6495, 0) projected
  line L124 (250.6495, 0) -> (250.6495, 16.325) projected
  line L125 (250.6495, 16.325) -> (253.1495, 16.325) projected
  arc A4 (253.1495, 16.325) -> (254.1495, 17.325) centre (253.1495, 17.325) ccw projected
  line L126 (254.1495, 17.325) -> (254.1495, 35.325) projected
  arc A5 (254.1495, 35.325) -> (253.1495, 36.325) centre (253.1495, 35.325) ccw projected
  line L127 (253.1495, 36.325) -> (250.6495, 36.325) projected
  line L128 (250.6495, 36.325) -> (250.6495, 77.7) projected
  line L129 (250.6495, 77.7) -> (234.3245, 77.7) projected
  line L130 (234.3245, 77.7) -> (234.3245, 80.2) projected
  arc A6 (234.3245, 80.2) -> (233.3245, 81.2) centre (233.3245, 80.2) ccw projected
  line L131 (233.3245, 81.2) -> (215.3245, 81.2) projected
  arc A7 (215.3245, 81.2) -> (214.3245, 80.2) centre (215.3245, 80.2) ccw projected
  line L132 (214.3245, 80.2) -> (214.3245, 77.7) projected
  line L133 (214.3245, 77.7) -> (177.1745, 77.7) projected
  line L134 (177.1745, 77.7) -> (177.1745, 80.2) projected
  arc A8 (177.1745, 80.2) -> (176.1745, 81.2) centre (176.1745, 80.2) ccw projected
  line L135 (176.1745, 81.2) -> (158.1745, 81.2) projected
  arc A9 (158.1745, 81.2) -> (157.1745, 80.2) centre (158.1745, 80.2) ccw projected
  line L136 (157.1745, 80.2) -> (157.1745, 77.7) projected
  line L137 (157.1745, 77.7) -> (115.7995, 77.7) projected
  line L138 (115.7995, 77.7) -> (115.7995, 57.9) projected
  arc A10 (103.237, -3.5) -> (104.237, -2.5) centre (103.237, -2.5) ccw projected
  line L139 (104.237, -2.5) -> (104.237, 0) projected
  line L140 (104.237, 0) -> (120.562, 0) projected
  line L141 (120.562, 0) -> (120.562, 19.05) projected
  line L142 (120.562, 19.05) -> (130.0875, 19.05) projected
  line L143 (130.0875, 19.05) -> (130.0875, 39.6) projected
  line L144 (130.0875, 39.6) -> (120.5625, 39.6) projected
  line L145 (120.5625, 39.6) -> (120.5625, 58.65) projected
  line L146 (120.5625, 58.65) -> (115.8, 58.65) projected
  line L147 (115.8, 58.65) -> (115.8, 77.7) projected
  line L148 (115.8, 77.7) -> (75.6625, 77.7) projected
  line L149 (75.6625, 77.7) -> (75.6625, 80.2) projected
  arc A11 (75.6625, 80.2) -> (74.6625, 81.2) centre (74.6625, 80.2) ccw projected
  line L150 (74.6625, 81.2) -> (56.6625, 81.2) projected
  arc A12 (56.6625, 81.2) -> (55.6625, 80.2) centre (56.6625, 80.2) ccw projected
  line L151 (55.6625, 80.2) -> (55.6625, 77.7) projected
  line L152 (55.6625, 77.7) -> (36.325, 77.7) projected
  line L153 (36.325, 77.7) -> (36.325, 80.2) projected
  arc A13 (36.325, 80.2) -> (35.325, 81.2) centre (35.325, 80.2) ccw projected
  line L154 (35.325, 81.2) -> (17.325, 81.2) projected
  arc A14 (17.325, 81.2) -> (16.325, 80.2) centre (17.325, 80.2) ccw projected
  line L155 (16.325, 80.2) -> (16.325, 77.7) projected
  line L156 (16.325, 77.7) -> (0, 77.7) projected
  line L157 (0, 77.7) -> (0, 61.375) projected
  line L158 (0, 61.375) -> (-2.5, 61.375) projected
  arc A15 (-2.5, 61.375) -> (-3.5, 60.375) centre (-2.5, 60.375) ccw projected
  line L159 (-3.5, 60.375) -> (-3.5, 42.375) projected
  arc A16 (-3.5, 42.375) -> (-2.5, 41.375) centre (-2.5, 42.375) ccw projected
  line L160 (-2.5, 41.375) -> (0, 41.375) projected
  line L161 (0, 41.375) -> (0, 0) projected
  line L162 (0, 0) -> (16.325, 0) projected
  line L163 (16.325, 0) -> (16.325, -2.5) projected
  arc A17 (16.325, -2.5) -> (17.325, -3.5) centre (17.325, -2.5) ccw projected
  line L164 (17.325, -3.5) -> (35.325, -3.5) projected
  arc A18 (35.325, -3.5) -> (36.325, -2.5) centre (35.325, -2.5) ccw projected
  line L165 (36.325, -2.5) -> (36.325, 0) projected
  line L166 (36.325, 0) -> (84.237, 0) projected
  line L167 (84.237, 0) -> (84.237, -2.5) projected
  arc A19 (84.237, -2.5) -> (85.237, -3.5) centre (85.237, -2.5) ccw projected
  line L168 (85.237, -3.5) -> (103.237, -3.5) projected
  line L169 (88.1304, 17.275) -> (108.6315, 17.275) projected
  line L170 (108.6315, 17.275) -> (108.6315, 18.2451) projected
  line L171 (108.6315, 18.2451) -> (111.9306, 18.2451) projected
  line L172 (111.9306, 18.2451) -> (111.9306, 17.275) projected
  line L173 (111.9306, 17.275) -> (114.4058, 17.275) projected
  line L174 (114.4058, 17.275) -> (114.4058, 3.9957) projected
  line L175 (114.4058, 3.9957) -> (105.3807, 3.9957) projected
  line L176 (105.3807, 3.9957) -> (105.3807, 3.2757) projected
  line L177 (105.3807, 3.2757) -> (91.3812, 3.2757) projected
  line L178 (91.3812, 3.2757) -> (91.3812, 3.9957) projected
  line L179 (91.3812, 3.9957) -> (82.3562, 3.9957) projected
  line L180 (82.3562, 3.9957) -> (82.3562, 17.275) projected
  line L181 (82.3562, 17.275) -> (84.8314, 17.275) projected
  line L182 (84.8314, 17.275) -> (84.8314, 18.2451) projected
  line L183 (84.8314, 18.2451) -> (88.1304, 18.2451) projected
  line L184 (88.1304, 18.2451) -> (88.1304, 17.275) projected
  line L185 (3.275, 60.425) -> (3.275, 74.425) projected
  line L186 (3.275, 74.425) -> (17.275, 74.425) projected
  line L187 (17.275, 74.425) -> (17.275, 60.425) projected
  line L188 (17.275, 60.425) -> (3.275, 60.425) projected
  line L189 (22.325, 60.425) -> (22.325, 74.425) projected
  line L190 (22.325, 74.425) -> (36.325, 74.425) projected
  line L191 (36.325, 74.425) -> (36.325, 60.425) projected
  line L192 (36.325, 60.425) -> (22.325, 60.425) projected
  line L193 (41.375, 60.425) -> (41.375, 74.425) projected
  line L194 (41.375, 74.425) -> (55.375, 74.425) projected
  line L195 (55.375, 74.425) -> (55.375, 60.425) projected
  line L196 (55.375, 60.425) -> (41.375, 60.425) projected
  line L197 (60.425, 60.425) -> (60.425, 74.425) projected
  line L198 (60.425, 74.425) -> (74.425, 74.425) projected
  line L199 (74.425, 74.425) -> (74.425, 60.425) projected
  line L200 (74.425, 60.425) -> (60.425, 60.425) projected
  line L201 (79.475, 60.425) -> (79.475, 74.425) projected
  line L202 (79.475, 74.425) -> (93.475, 74.425) projected
  line L203 (93.475, 74.425) -> (93.475, 60.425) projected
  line L204 (93.475, 60.425) -> (79.475, 60.425) projected
  line L205 (98.525, 60.425) -> (98.525, 74.425) projected
  line L206 (98.525, 74.425) -> (112.525, 74.425) projected
  line L207 (112.525, 74.425) -> (112.525, 60.425) projected
  line L208 (112.525, 60.425) -> (98.525, 60.425) projected
  line L209 (27.0875, 41.375) -> (27.0875, 55.375) projected
  line L210 (27.0875, 55.375) -> (41.0875, 55.375) projected
  line L211 (41.0875, 55.375) -> (41.0875, 41.375) projected
  line L212 (41.0875, 41.375) -> (27.0875, 41.375) projected
  line L213 (46.1375, 41.375) -> (46.1375, 55.375) projected
  line L214 (46.1375, 55.375) -> (60.1375, 55.375) projected
  line L215 (60.1375, 55.375) -> (60.1375, 41.375) projected
  line L216 (60.1375, 41.375) -> (46.1375, 41.375) projected
  line L217 (65.1875, 41.375) -> (65.1875, 55.375) projected
  line L218 (65.1875, 55.375) -> (79.1875, 55.375) projected
  line L219 (79.1875, 55.375) -> (79.1875, 41.375) projected
  line L220 (79.1875, 41.375) -> (65.1875, 41.375) projected
  line L221 (84.2375, 41.375) -> (84.2375, 55.375) projected
  line L222 (84.2375, 55.375) -> (98.2375, 55.375) projected
  line L223 (98.2375, 55.375) -> (98.2375, 41.375) projected
  line L224 (98.2375, 41.375) -> (84.2375, 41.375) projected
  line L225 (103.2875, 41.375) -> (103.2875, 55.375) projected
  line L226 (103.2875, 55.375) -> (117.2875, 55.375) projected
  line L227 (117.2875, 55.375) -> (117.2875, 41.375) projected
  line L228 (117.2875, 41.375) -> (103.2875, 41.375) projected
  line L229 (36.6125, 22.325) -> (36.6125, 36.325) projected
  line L230 (36.6125, 36.325) -> (50.6125, 36.325) projected
  line L231 (50.6125, 36.325) -> (50.6125, 22.325) projected
  line L232 (50.6125, 22.325) -> (36.6125, 22.325) projected
  line L233 (55.6625, 22.325) -> (55.6625, 36.325) projected
  line L234 (55.6625, 36.325) -> (69.6625, 36.325) projected
  line L235 (69.6625, 36.325) -> (69.6625, 22.325) projected
  line L236 (69.6625, 22.325) -> (55.6625, 22.325) projected
  line L237 (74.7125, 22.325) -> (74.7125, 36.325) projected
  line L238 (74.7125, 36.325) -> (88.7125, 36.325) projected
  line L239 (88.7125, 36.325) -> (88.7125, 22.325) projected
  line L240 (88.7125, 22.325) -> (74.7125, 22.325) projected
  line L241 (93.7625, 22.325) -> (93.7625, 36.325) projected
  line L242 (93.7625, 36.325) -> (107.7625, 36.325) projected
  line L243 (107.7625, 36.325) -> (107.7625, 22.325) projected
  line L244 (107.7625, 22.325) -> (93.7625, 22.325) projected
  line L245 (112.8125, 22.325) -> (112.8125, 36.325) projected
  line L246 (112.8125, 36.325) -> (126.8125, 36.325) projected
  line L247 (126.8125, 36.325) -> (126.8125, 22.325) projected
  line L248 (126.8125, 22.325) -> (112.8125, 22.325) projected
  line L249 (5.6562, 41.375) -> (5.6562, 55.375) projected
  line L250 (5.6562, 55.375) -> (19.6562, 55.375) projected
  line L251 (19.6562, 55.375) -> (19.6562, 41.375) projected
  line L252 (19.6562, 41.375) -> (5.6562, 41.375) projected
  line L253 (5.6562, 3.275) -> (5.6562, 17.275) projected
  line L254 (5.6562, 17.275) -> (19.6562, 17.275) projected
  line L255 (19.6562, 17.275) -> (19.6562, 3.275) projected
  line L256 (19.6562, 3.275) -> (5.6562, 3.275) projected
  line L257 (31.85, 3.275) -> (31.85, 17.275) projected
  line L258 (31.85, 17.275) -> (45.85, 17.275) projected
  line L259 (45.85, 17.275) -> (45.85, 3.275) projected
  line L260 (45.85, 3.275) -> (31.85, 3.275) projected
  line L261 (58.0437, 3.275) -> (58.0437, 17.275) projected
  line L262 (58.0437, 17.275) -> (72.0437, 17.275) projected
  line L263 (72.0437, 17.275) -> (72.0437, 3.275) projected
  line L264 (72.0437, 3.275) -> (58.0437, 3.275) projected
  line L265 (10.4187, 22.325) -> (10.4187, 36.325) projected
  line L266 (10.4187, 36.325) -> (24.4187, 36.325) projected
  line L267 (24.4187, 36.325) -> (24.4187, 22.325) projected
  line L268 (24.4187, 22.325) -> (10.4187, 22.325) projected
  point P0 (115.8, 77.7)
extrude "Extrusion3" cut sketch "Sketch3" against normal blind 10 contours L138 L146 L145 L108 | L144 L143 L111 L110 | L143 L142 L114 L113
fillet "Fillet3" radius 1 7 edges at (115.8, 77.7, 0.7) (120.5625, 57.9, 0.7) (130.0875, 38.85, 0.7) (130.0875, 19.8, 0.7) (120.562, 0, 0.7) (0, 0, 0.7) (0, 77.7, 0.7)
body "Solid1"
